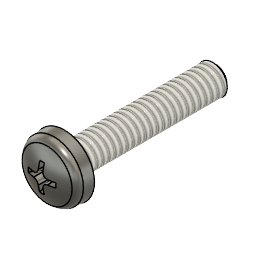
drone-fusion (Autodesk Fusion 360 archive; units mm, degrees)
design "Pan Head Screw JIS B 1111 - M2 x 10 - H Steel 4.6 Plain"
description: Pan Head Screw JIS B 1111 - M2 x 10 - H
part number: PHS JIS B 1111 - M2 x 10 - H Steel 4.6 Plain
Autodesk Fusion 360 part; units mm, degrees
sketch "Sketch1" plane through (0, 0, 0) normal (0, 1, 0) x (1, 0, 0)
  line L0 (-1, 0.8) -> (-1, 10)
  line L1 (-1, 10) -> (0, 10)
  line L2 (0, 10) -> (0, -1.6)
  line L3 (-0.8773, 0) -> (-2, 0)
  arc A0 (-1.9157, -0.9632) -> (0, -1.6) centre (0, 1.6) ccw
  line L4 (-1, 0.8) -> (-0.8772, 0.5368)
  line L5 (-0.8772, 0.5368) -> (-0.8773, 0)
  line L6 (-2, 0) -> (-1.9157, -0.9632)
  dimension "d9" = 2
  dimension "d66" = 4
  dimension "d75" = 1.7545
  dimension "d77" = 0.8
  dimension "d78" = 155
  dimension "d103" = 5
  dimension "d111" = 1.6
  dimension "d112" = 10
  constraint perpendicular L0 L1
  constraint collinear origin L2.end L1.end
  constraint perpendicular L0 L3
  constraint coincident origin L3
  constraint vertical L0
  constraint vertical L2
  constraint coincident L2 A0.centre
  constraint perpendicular L3 L5
  constraint coincident L3.start L5.end
  measures "d77" distance of L3 L0.start
  measures "d78" angle of L0 L4
  measures "d103" angle of L2 L6
  measures "d111" distance of L2.end L3
  measures "d112" distance of origin L1
revolve "Revolve1" add sketch "Sketch1" angle 360 about axis through (0, 0, -10) along (0, 0, 1) makes body 1
ref_plane "WorkPlane1" through (0, 0, 1.6) normal (0, 0, 1) x (1, 0, 0)
sketch "Sketch2" plane through (0, 0, 1.6) normal (0, 0, 1) x (1, 0, 0)
  line L0 (-0.155, 0.155) -> (-1, 0.155)
  line L1 (-0.155, -0.155) -> (-1, -0.155)
  line L2 (-1, 0.155) -> (-1, -0.155)
  line L3 (-0.155, -0.155) -> (-0.155, -1)
  line L4 (-0.155, -1) -> (0.155, -1)
  line L5 (0.155, -0.155) -> (0.155, -1)
  line L6 (0.155, -0.155) -> (1, -0.155)
  line L7 (1, -0.155) -> (1, 0.155)
  line L8 (0.155, 0.155) -> (1, 0.155)
  line L9 (0.155, 0.155) -> (0.155, 1)
  line L10 (0.155, 1) -> (-0.155, 1)
  line L11 (-0.155, 0.155) -> (-0.155, 1)
  dimension "d105" = 0.31
  dimension "d107" = 360
  dimension "d108" = 2
  constraint perpendicular L1 L2
  constraint vertical L0.start L1.start
  constraint horizontal L1
  constraint coincident L8.start L9.start
  measures "d105" distance of L0 L1
  measures "d108" distance of L2 L7
extrude "Extrude1" add sketch "Sketch2" against normal blind 1.2 draft -4 separate body makes body 2
draft "Draft1" angle -30 neutral plane through (0, 0, 1.6) pull (0, 0, 1) 4 faces at (-0.972, -0.0237, 1.2) (-0.0237, -0.972, 1.2) (0.972, -0.0237, 1.2) (-0.0237, 0.972, 1.2) on bodies 2
fillet "Fillet3" radius 0.31 4 edges at (0.113, 0.113, 1) (-0.113, 0.113, 1) (0.113, -0.113, 1) (-0.113, -0.113, 1) on bodies 2
combine "Combine1" operation cut target body 1 tool bodies 2
fillet "Fillet4" radius 0.6 1 edges at (-1.7861, 0.6928, 0.9632) on bodies 1
thread "Thread1" "ISO Metric profile 2.0 M2x0.4 M2x0.4 6g" major diameter 1.9335 minor diameter 1.478 pitch 0.4 angle 60 resizes the face on face at (-0.995, 0.0996, -6.9333) on bodies 1
fillet "Fillet5" radius 0.8 1 edges at (-0.8179, 0.3172, 0) on bodies 1
sketch "Sketch5" plane through (0, 0, 0) normal (0, 1, 0) x (1, 0, 0)
  line L0 (-1.02, 10) -> (-1.02, 9.7546)
  line L1 (-1.02, 9.7546) -> (-0.7546, 10)
  line L2 (0, 10) -> (0, -1.6)
  line L3 (-1.02, 10) -> (0, 10)
  dimension "d114" = 0.2454
  dimension "d115" = 1.02
  dimension "d116" = 0.2654
  constraint coincident L2.start L3.end
  constraint perpendicular L2 L3
  constraint coincident L1.end L3
  constraint perpendicular L0 L3
  measures "d114" distance of L0.end L3
  measures "d115" distance of L0 L2.start
  measures "d116" distance of L0 L1.end
revolve "Revolve2" cut sketch "Sketch5" angle 360 about axis through (0, 0, -10) along (0, 0, 1) bodies 1
equation "d9 = adsk_nomdia"
equation "adsk_nomlen = 10.00 mm"
equation "adsk_headh = 1.60 mm"
equation "adsk_headdia = 4.00 mm"
equation "adsk_nomdia = 2.00 mm"
equation "adsk_phildia = 2.00 mm"
equation "d31 = -adsk_phildepth"
equation "adsk_philwidth = 0.31 mm"
equation "adsk_phildepth = 1.20 mm"
equation "d66 = adsk_headdia"
equation "d71 = adsk_headh"
equation "adsk_thrlen = 9.20 mm"
equation "d75 = adsk_shnkdia"
equation "adsk_shnkdia = 1.7545 mm"
equation "d77 = adsk_nomlen - adsk_thrlen"
equation "adsk_endpointdia = 1.50924 mm"
equation "adsk_startlen = 0.24538 mm"
equation "adsk_ovalrad = 3.20 mm"
equation "adsk_headtoprad = adsk_nomdia * 0.3"
equation "adsk_midfillet = 0.80 mm"
equation "d98 = adsk_midfillet"
equation "adsk_headang = 5.00 deg"
equation "d102 = adsk_headtoprad"
equation "d103 = adsk_headang"
equation "d105 = adsk_philwidth"
equation "d108 = adsk_phildia"
equation "d110 = adsk_philwidth"
equation "d111 = adsk_headh"
equation "d112 = adsk_nomlen"
equation "d113 = ( adsk_nomlen + adsk_headh ) - ( adsk_ovalrad )"
equation "d114 = adsk_startlen"
equation "d115 = adsk_nomdia * 0.51"
equation "d116 = ( adsk_nomdia * 0.51 ) - ( adsk_endpointdia / 2 )"
